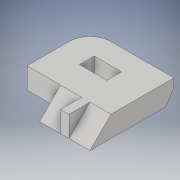
# Autodesk Inventor part: T2 Part I
Saved by Autodesk Inventor 2018 (Build 220112000, 112)
## iProperties
Created: 2018-09-15
Part Number: T2 Part I
Material: Generic
Document SubType Name: Modeling
Designer: Saon
Density: 1 g/cm^3
Appearance: Default
Author: Saon
Autodesk Inventor part; units mm, degrees
ref_plane "YZ Plane" through (0, 0, 0) normal (1, 0, 0) x (0, 1, 0)
ref_plane "XZ Plane" through (0, 0, 0) normal (0, 1, 0) x (-1, 0, 0)
ref_plane "XY Plane" through (0, 0, 0) normal (0, 0, 1) x (1, 0, 0)
sketch "Sketch1" plane through (0, 0, 0) normal (0, 1, 0) x (-1, 0, 0)
  line L0 (0, 0) -> (10, 0)
  line L1 (10, 0) -> (14, 0)
  line L2 (14, 0) -> (24, 0)
  line L3 (24, 0) -> (24, -10)
  line L4 (24, -10) -> (40, -10)
  line L5 (0, 0) -> (0, -40)
  line L6 (0, -40) -> (30, -40)
  line L7 (40, -30) -> (40, -10)
  arc A0 (30, -40) -> (40, -30) centre (30, -30) ccw
  line L8 (28, -30) -> (15, -30)
  line L9 (15, -30) -> (15, -23)
  line L10 (15, -23) -> (28, -23)
  line L11 (28, -23) -> (28, -30)
  dimension "d0" = 10
  dimension "d1" = 4
  dimension "d2" = 10
  dimension "d3" = 10
  dimension "d4" = 16
  dimension "d5" = 40
  dimension "d6" = 10
  dimension "d7" = 13
  dimension "d8" = 7
  dimension "d9" = 13
  dimension "d10" = 12
  constraints: 24 end point, 5 perpendicular, 2 horizontal, 2 parallel, 2 point on circle, 2 point on line, 2 tangent, 1 centre point, 1 vertical
  measures "d0" distance of L0.start L0.end
  measures "d1" distance of L0.end L1.end
  measures "d2" distance of L1.end L2.end
  measures "d3" distance of L2.end L3.end
  measures "d4" distance of L3.end L4.end
  measures "d5" distance of L0.start L5.end
  measures "d6" radius of A0
  measures "d7" distance of L9.end L10.end
  measures "d8" distance of L8.end L9.end
  measures "d9" distance between parallel lines of L10 L4
  measures "d10" distance between parallel lines of L7 L11
extrude "Extrusion1" add sketch "Sketch1" along normal blind 10
sketch "Sketch2" plane through (-24, 0, -10) normal (-1, 0, 0) x (0, 0, 1)
  line L0 (0, 0) -> (0, 10) projected
  line L1 (-30, 0) -> (10, 0) projected
  line L2 (0, 10) -> (10, 0)
  line L3 (10, 0) -> (10, 10)
  line L4 (10, 10) -> (0, 10)
  constraints: 6 end point, 2 perpendicular
extrude "Extrusion2" cut sketch "Sketch2" against normal blind 10 contours L4 L3 L2
sketch "Sketch3" plane through (0, 0, 0) normal (1, 0, 0) x (0, 0, -1)
  line L0 (0, 0) -> (10, 10) projected
  line L1 (0, 0) -> (0, 10) projected
  line L2 (30, 10) -> (10, 10) projected
  line L3 (0, 0) -> (10, 10)
  line L4 (10, 10) -> (0, 10)
  line L5 (0, 10) -> (0, 0)
  constraints: 6 end point, 1 horizontal, 1 perpendicular
extrude "Extrusion3" cut sketch "Sketch3" against normal blind 10
sketch "Sketch4" plane through (0, 0, -40) normal (1, 0, 0) x (0, 0, -1)
  line L0 (0, 0) -> (-4, 0)
  line L1 (-10, 0) -> (0, 0) projected
  line L2 (0, 0) -> (0, 10) projected
  line L3 (0, 10) -> (0, 6)
  line L4 (0, 6) -> (-4, 0)
  line L5 (0, 6) -> (0, 0)
  point P0 (-40, 0)
  dimension "d17" = 4
  dimension "d18" = 4
  constraints: 8 end point, 2 point on line, 1 vertical
  measures "d17" distance of L0.start L0.end
  measures "d18" distance of L2.end L3.end
extrude "Extrusion4" cut sketch "Sketch4" against normal blind 6
body "Solid1"
